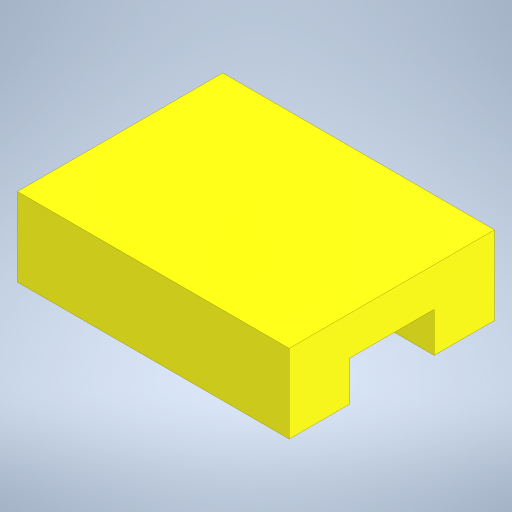
# Autodesk Inventor part: MGN7C_slider
Saved by Autodesk Inventor 2024 (Build 280153000, 153)
## iProperties
Created: 2023-08-26
Part Number: MGN7C_slider
Material: ABS Plastic
Document SubType Name: Modeling
Designer: l1534
Density: 1.06 g/cm^3
Appearance: Smooth - Yellow
Author: l1534
Autodesk Inventor part; units mm, degrees
ref_plane "YZ Plane" through (0, 0, 0) normal (1, 0, 0) x (0, 1, 0)
ref_plane "XZ Plane" through (0, 0, 0) normal (0, 1, 0) x (-1, 0, 0)
ref_plane "XY Plane" through (0, 0, 0) normal (0, 0, 1) x (1, 0, 0)
sketch "Sketch1" plane through (0, 0, 0) normal (1, 0, 0) x (0, 1, 0)
  line L0 (5.7363, 8.6903) -> (-0.7637, 8.6903)
  line L1 (-0.7637, 8.6903) -> (-0.7637, 3.6903)
  line L2 (-0.7637, 3.6903) -> (2.5363, 3.6903)
  line L3 (2.5363, 3.6903) -> (2.5363, -3.3097)
  line L4 (2.5363, -3.3097) -> (-0.7637, -3.3097)
  line L5 (-0.7637, -3.3097) -> (-0.7637, -8.3097)
  line L6 (-0.7637, -8.3097) -> (5.7363, -8.3097)
  line L7 (5.7363, -8.3097) -> (5.7363, 8.6903)
  point P0 (0, 0)
  dimension "d0" = 17
  dimension "d1" = 3.3
  dimension "d2" = 6.5
  dimension "d3" = 5
  dimension "d4" = 7
  constraints: 16 end point, 6 perpendicular, 2 point on line, 1 horizontal
  measures "d0" distance of L6.end L0.start
  measures "d1" distance of L3.end L4.end
  measures "d2" distance of L5.end L6.end
  measures "d3" distance of L4.end L5.end
  measures "d4" distance of L2.end L3.end
extrude "Extrusion1" add sketch "Sketch1" along normal blind 22.5
body "Solid1"
